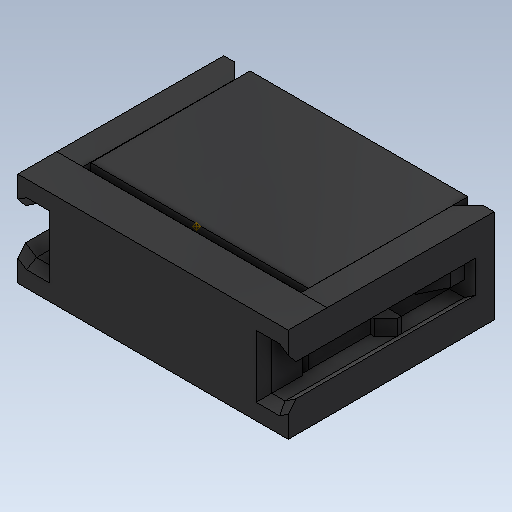
# Autodesk Inventor part: ribbon cable connector
Saved by Autodesk Inventor 2020.1 (Build 241239000, 239)
## iProperties
Created: 2007-05-08
Part Number: ribbon cable connector
Document SubType Name: Modeling
Designer: floress
Density: 1 g/cm^3
Categories: <MemberInstance><Categories><Category DisplayName="" Mnemonic="CABLEANDHARNESS" InternalName="e4a7e005-5e42-4d16-b293-125e7f0d0512"><Category DisplayName="" Mnemonic="CONNECTORS" InternalName="6f634eba-a678-4820-a31d-2c2d5ee6728e"><CategoryParameter DisplayName="" Mnemonic="REFDES" InternalName="c3740e8c-60ab-4d5d-8584-52b73222f2f0"/><Category DisplayName="" Mnemonic="RIBBONCABLE" InternalName="27621a3d-53ec-49ed-8225-e2ac65e8eb52"/></Category></Category></Categories><FamilyTemplate><FamilyTemplateParameters></FamilyTemplateParameters></FamilyTemplate><CategoryParameterMap><ParamToTemplateMap><ParamToTemplate CategoryParameter="//CategoryParameter[@InternalName='c3740e8c-60ab-4d5d-8584-52b73222f2f0']" ConstantValue=""/></ParamToTemplateMap></CategoryParameterMap></MemberInstance>
Material: Generic
Appearance: Dark Gray
Author: floress
Autodesk Inventor part; units mm, degrees
ref_plane "YZ Plane" through (0, 0, 0) normal (1, 0, 0) x (0, 1, 0)
ref_plane "XZ Plane" through (0, 0, 0) normal (0, 1, 0) x (-1, 0, 0)
sketch "Sketch1" plane through (0, 0, 0) normal (0, 0, 1) x (1, 0, 0)
  line L0 (6.98, -3) -> (-6.98, -3)
  line L1 (-6.23, -1.5) -> (-6.23, -2.1)
  line L2 (-6.98, -3) -> (-6.98, -2.1)
  line L3 (-6.23, -2.1) -> (-6.98, -2.1)
  line L4 (-6.98, -1.5) -> (-6.23, -1.5)
  line L5 (-6.98, -1.5) -> (-6.98, 3)
  line L6 (6.23, 1.5) -> (6.23, 2.1)
  line L7 (6.98, 1.5) -> (6.98, -3)
  line L8 (6.98, 1.5) -> (6.23, 1.5)
  line L9 (6.23, 2.1) -> (6.98, 2.1)
  line L10 (6.98, 3) -> (6.98, 2.1)
  line L11 (0, 3) -> (0, -3) construction
  line L12 (-6.98, 3) -> (6.98, 3)
  point P0 (0, 0)
  point P1 (0, 0)
  constraints: 26 end point, 8 parallel, 3 midpoint, 3 perpendicular, 2 horizontal, 1 coincident
extrude "Extrusion1" add sketch "Sketch1" along normal blind 10.2
sketch "Sketch2" plane through (-6.98, -3, 0) normal (0, -1, 0) x (1, 0, 0)
  line L0 (5.18, 3.6) -> (8.78, 3.6)
  line L1 (8.78, 3.6) -> (8.78, 0.5)
  line L2 (8.28, 0) -> (5.68, 0)
  line L3 (5.18, 0.5) -> (5.18, 3.6)
  line L4 (5.18, 0.5) -> (5.68, 0)
  line L5 (8.78, 0.5) -> (8.28, 0)
  point P0 (6.98, 0)
  constraints: 12 end point, 2 parallel, 1 horizontal, 1 midpoint, 1 perpendicular
extrude "Extrusion2" add sketch "Sketch2" along normal blind 1
sketch "Sketch3" plane through (0, 0, 0) normal (0, 1, 0) x (-1, 0, 0)
  line L0 (-6.98, 3.6) -> (-7.23, 3.6)
  line L1 (-7.98, 2.1) -> (-7.98, 1.22)
  line L2 (-7.98, 1.22) -> (-6.98, 1.22)
  line L3 (-6.98, 1.22) -> (-6.98, 3.6)
  line L4 (6.98, 10.2) -> (-6.98, 10.2)
  line L5 (0, 10.2) -> (0, 0)
  line L6 (-6.98, 0) -> (6.98, 0)
  line L7 (-7.23, 3.6) -> (-7.98, 2.1)
  line L8 (6.98, 3.6) -> (7.23, 3.6)
  line L9 (7.98, 2.1) -> (7.98, 1.22)
  line L10 (7.98, 1.22) -> (6.98, 1.22)
  line L11 (6.98, 1.22) -> (6.98, 3.6)
  line L12 (7.23, 3.6) -> (7.98, 2.1)
  constraints: 26 end point, 5 symmetric about line, 2 midpoint, 2 parallel, 2 perpendicular, 1 horizontal
extrude "Extrusion3" add sketch "Sketch3" along normal mid plane 1
sketch "Sketch4" plane through (0, -0.5, 0) normal (0, -1, 0) x (1, 0, 0)
  line L0 (6.98, 3.6) -> (7.23, 3.6)
  line L1 (6.98, 6.263) -> (7.23, 6.263)
  line L2 (7.98, 5.513) -> (7.98, 5.263)
  line L3 (7.98, 5.263) -> (6.98, 5.263)
  line L4 (6.98, 5.263) -> (6.98, 6.263)
  line L5 (-6.98, 10.2) -> (6.98, 10.2)
  line L6 (7.23, 6.263) -> (7.98, 5.513)
  line L7 (-6.98, 5.263) -> (-6.98, 6.263)
  line L8 (-6.98, 6.263) -> (-7.23, 6.263)
  line L9 (-7.23, 6.263) -> (-7.98, 5.513)
  line L10 (-7.98, 5.513) -> (-7.98, 5.263)
  line L11 (-7.98, 5.263) -> (-6.98, 5.263)
  point P0 (0, 10.2)
  constraints: 24 end point, 2 parallel, 1 horizontal, 1 midpoint, 1 perpendicular
extrude "Extrusion4" add sketch "Sketch4" along normal blind 1
sketch "Sketch5" plane through (0, 0.5, 0) normal (0, 1, 0) x (1, 0, 0)
  line L0 (7.23, -3.6) -> (6.98, -3.6)
  line L1 (7.23, -6.263) -> (6.98, -6.263)
  line L2 (6.98, -6.263) -> (6.98, -5.263)
  line L3 (6.98, -5.263) -> (7.98, -5.263)
  line L4 (7.98, -5.263) -> (7.98, -5.513)
  line L5 (6.98, -10.2) -> (-6.98, -10.2)
  line L6 (1.3, 0) -> (-1.3, 0)
  line L7 (0, 0) -> (0, -10.2)
  line L8 (7.23, -6.263) -> (7.98, -5.513)
  line L9 (-6.98, -6.263) -> (-6.98, -5.263)
  line L10 (-7.23, -6.263) -> (-6.98, -6.263)
  line L11 (-7.23, -6.263) -> (-7.98, -5.513)
  line L12 (-7.98, -5.263) -> (-7.98, -5.513)
  line L13 (-6.98, -5.263) -> (-7.98, -5.263)
  line L14 (6.98, -3.6) -> (6.98, -1.22)
  line L15 (7.98, -2.1) -> (7.23, -3.6)
  line L16 (7.98, -1.22) -> (7.98, -2.1)
  line L17 (6.98, -1.22) -> (7.98, -1.22)
  dimension "d35" = 1.663
  dimension "d36" = 13.96
  dimension "d37" = 1
  dimension "d38" = 1
  dimension "d39" = 0.25
  dimension "d40" = 0.25
  constraints: 36 end point, 5 symmetric about line, 2 midpoint, 2 parallel, 1 horizontal, 1 perpendicular
  measures "d35" distance between parallel lines of L0 L3
  measures "d36" diameter of L2 L7
  measures "d37" distance of L2.start L2.end
  measures "d38" distance of L2.end L4.start
  measures "d39" distance of L1.start L2.start
  measures "d40" distance of L4.start L8.end
extrude "Extrusion5" add sketch "Sketch5" along normal blind 1 contours L1 L2 L3 L4 L8 | L10 L11 L12 L13 L9
sketch "Sketch6" plane through (-6.98, -3, 10.2) normal (0, -1, 0) x (1, 0, 0)
  line L0 (0.5, -10.2) -> (2.5, -6.7359)
  line L1 (2.5, -6.7359) -> (4.5, -10.2)
  line L2 (0.5, -10.2) -> (4.5, -10.2)
  line L3 (5.68, -10.2) -> (5.18, -9.7)
  line L4 (5.18, -9.7) -> (5.18, -6.6)
  constraints: 10 end point, 2 equal length
extrude "Extrusion6" cut sketch "Sketch6" against normal blind 0.1
sketch "Sketch7" plane through (0, 0, 0) normal (0, 0, -1) x (-1, 0, 0)
  line L0 (6.98, 3) -> (6.98, -1.5)
  line L1 (4.705, 1.645) -> (5.455, 1.645)
  line L2 (5.455, 1.645) -> (5.455, 0.895)
  line L3 (5.455, 0.895) -> (4.705, 0.895)
  line L4 (4.705, 0.895) -> (4.705, 1.645)
  line L5 (4.705, -0.895) -> (5.455, -0.895)
  line L6 (5.455, -0.895) -> (5.455, -1.645)
  line L7 (5.455, -1.645) -> (4.705, -1.645)
  line L8 (4.705, -1.645) -> (4.705, -0.895)
  line L9 (5.08, 0.895) -> (5.08, -0.895) construction
  line L10 (6.48, -2.9) -> (6.48, -3)
  line L11 (6.98, -3) -> (6.48, -3)
  line L12 (6.98, -2.1) -> (6.98, -3)
  line L13 (6.23, -2.1) -> (6.98, -2.1)
  line L14 (6.23, -1.5) -> (6.23, -2.1)
  point P0 (5.08, 0)
  constraints: 30 end point, 7 equal length, 4 parallel, 3 midpoint, 3 perpendicular, 2 horizontal
extrude "Extrusion7" cut sketch "Sketch7" against normal blind 3
chamfer "Chamfer1" distance 0.5 angle 45 8 edges at (-4.705, 1.27, 0) (-5.08, 0.895, 0) (-5.455, 1.27, 0) (-5.08, 1.645, 0) (-4.705, -1.27, 0) (-5.08, -1.645, 0) (-5.455, -1.27, 0) (-5.08, -0.895, 0)
pattern_linear "Rectangular Pattern1" count 5 spacing 2.54 along (1, 0, 0) of "Extrusion7", "Chamfer1"
ref_plane "Work Plane1" through (0, 0, 10.7) normal (0, 0, 1) x (1, 0, 0)
sketch "Sketch8" plane through (0, 0, 10.7) normal (0, 0, 1) x (1, 0, 0)
  line L0 (-7.9608, -1.4995) -> (-7.11, -1.4995)
  line L1 (-8.665, -1.03) -> (-7.9608, -1.4995)
  line L2 (-8.665, -3.03) -> (-8.665, -1.03)
  line L3 (8.665, -3.03) -> (-8.665, -3.03)
  line L4 (-8.665, 3.03) -> (8.665, 3.03)
  line L5 (-7.11, -1.4995) -> (-7.11, 1.4995)
  line L6 (-6.98, 3) -> (6.98, 3)
  line L7 (-6.98, -1.5) -> (-6.98, 3)
  line L8 (-6.23, -1.5) -> (-6.98, -1.5)
  line L9 (-6.23, -2.1) -> (-6.23, -1.5)
  line L10 (-6.98, -2.1) -> (-6.23, -2.1)
  line L11 (-6.98, -3) -> (-6.98, -2.1)
  line L12 (6.98, -3) -> (-6.98, -3)
  line L13 (6.98, 1.5) -> (6.98, -3)
  line L14 (6.23, 1.5) -> (6.98, 1.5)
  line L15 (6.23, 2.1) -> (6.23, 1.5)
  line L16 (6.98, 2.1) -> (6.23, 2.1)
  line L17 (6.98, 3) -> (6.98, 2.1)
  line L18 (0, 3) -> (0, -3)
  line L19 (-8.665, 1.03) -> (-7.9608, 1.4995)
  line L20 (-8.665, 3.03) -> (-8.665, 1.03)
  line L21 (-7.9608, 1.4995) -> (-7.11, 1.4995)
  line L22 (8.665, 3.03) -> (8.665, 1.03)
  line L23 (8.665, 1.03) -> (7.9608, 1.4995)
  line L24 (7.9608, 1.4995) -> (7.11, 1.4995)
  line L25 (7.11, -1.4995) -> (7.11, 1.4995)
  line L26 (7.9608, -1.4995) -> (7.11, -1.4995)
  line L27 (8.665, -1.03) -> (7.9608, -1.4995)
  line L28 (8.665, -3.03) -> (8.665, -1.03)
  point P0 (0, 0)
  point P1 (0, 0)
  point P2 (-8.665, -2.03)
  point P3 (-7.11, 0)
  point P4 (0, 0)
  constraints: 58 end point, 6 symmetric about line, 5 midpoint, 3 parallel, 3 perpendicular, 1 coincident, 1 horizontal, 1 horizontal alignment
extrude "Extrusion8" add sketch "Sketch8" along normal blind 2.5 contours L0 L5 L21 L19 L20 L4 L22 L23 L24 L25 L26 L27 L28 L3 L2 L1 | L6 L18 L12 L11 L10 L9 L8 L7 | L6 L17 L16 L15 L14 L13 L12 L18
sketch "Sketch9" plane through (0, 0, 10.7) normal (0, 0, -1) x (-1, 0, 0)
  line L0 (-8.665, 3.03) -> (-8.665, 1.03)
  line L1 (8.665, 1.03) -> (8.665, 3.03)
  line L2 (7.9608, 1.4995) -> (8.665, 1.03)
  line L3 (7.11, 1.4995) -> (7.9608, 1.4995)
  line L4 (7.9608, -1.4995) -> (7.11, -1.4995)
  line L5 (8.665, -1.03) -> (7.9608, -1.4995)
  line L6 (8.665, -3.03) -> (8.665, -1.03)
  line L7 (-8.665, -1.03) -> (-8.665, -3.03)
  line L8 (-7.9608, -1.4995) -> (-8.665, -1.03)
  line L9 (-7.11, -1.4995) -> (-7.9608, -1.4995)
  line L10 (-7.9608, 1.4995) -> (-7.11, 1.4995)
  line L11 (-8.665, 1.03) -> (-7.9608, 1.4995)
  line L12 (-6.99, 1.51) -> (-6.24, 1.51)
  line L13 (-6.24, 1.51) -> (-6.24, 2.09)
  line L14 (-6.24, 2.09) -> (-6.99, 2.09)
  line L15 (-6.99, 2.09) -> (-6.99, 3.03)
  line L16 (6.99, -2.09) -> (6.24, -2.09)
  line L17 (6.24, -2.09) -> (6.24, -1.51)
  line L18 (6.24, -1.51) -> (6.99, -1.51)
  line L19 (6.99, -3.03) -> (6.99, -2.09)
  line L20 (-7.11, -1.4995) -> (-6.99, -1.4995)
  line L21 (-7.11, 1.4995) -> (-6.99, 1.4995)
  line L22 (-6.99, -3.03) -> (-6.99, -1.4995)
  line L23 (-6.99, 1.4995) -> (-6.99, 1.51)
  line L24 (7.11, 1.4995) -> (6.99, 1.4995)
  line L25 (7.11, -1.4995) -> (6.99, -1.4995)
  line L26 (6.99, -1.51) -> (6.99, -1.4995)
  line L27 (6.99, 1.4995) -> (6.99, 3.03)
  line L28 (-8.665, 3.03) -> (-8.665, 1.03)
  line L29 (-8.665, 1.03) -> (-7.9608, 1.4995)
  line L30 (-7.9608, 1.4995) -> (-7.11, 1.4995)
  line L31 (-7.11, -1.4995) -> (-7.9608, -1.4995)
  line L32 (-7.9608, -1.4995) -> (-8.665, -1.03)
  line L33 (-8.665, -1.03) -> (-8.665, -3.03)
  line L34 (8.665, -3.03) -> (8.665, -1.03)
  line L35 (8.665, -1.03) -> (7.9608, -1.4995)
  line L36 (7.9608, -1.4995) -> (7.11, -1.4995)
  line L37 (7.11, 1.4995) -> (7.9608, 1.4995)
  line L38 (7.9608, 1.4995) -> (8.665, 1.03)
  line L39 (8.665, 1.03) -> (8.665, 3.03)
  line L40 (8.665, -3.03) -> (6.99, -3.03)
  line L41 (-8.665, -3.03) -> (-6.99, -3.03)
  line L42 (-8.665, 3.03) -> (-6.99, 3.03)
  line L43 (6.99, 3.03) -> (8.665, 3.03)
  constraints: 88 end point, 8 parallel, 6 perpendicular, 2 collinear, 2 horizontal
extrude "Extrusion9" add sketch "Sketch9" along normal blind 10.7
sketch "Sketch10" plane through (0, 0, 0) normal (0, 1, 0) x (-1, 0, 0)
  line L0 (-8.665, 0) -> (-6.99, 0)
  line L1 (-6.99, 0) -> (-6.99, 1.21)
  line L2 (-6.99, 1.21) -> (-8.665, 1.21)
  line L3 (-8.665, 1.21) -> (-8.665, 0)
  line L4 (6.99, 0) -> (6.99, 1.21)
  line L5 (6.99, 1.21) -> (8.665, 1.21)
  line L6 (8.665, 1.21) -> (8.665, 0)
  line L7 (8.665, 0) -> (6.99, 0)
  constraints: 16 end point, 2 parallel, 1 horizontal, 1 perpendicular
extrude "Extrusion10" add sketch "Sketch10" along normal mid plane 6.06
chamfer "Chamfer2" distance 1 angle 45 4 edges at (6.99, 2.56, 0) (6.99, -0.76, 0) (-6.99, 0.76, 0) (-6.99, -2.56, 0)
chamfer "Chamfer3" distance 1.749 angle 45 2 edges at (-6.24, -1.8, 0) (6.24, 1.8, 0)
chamfer "Chamfer4" distance 10.71 distance2 0.03 1 edges at (8.3275, -3.03, 0) measured on face at (2.33, -3.03, 12.3667)
chamfer "Chamfer5" distance 10.71 distance2 0.03 1 edges at (8.3275, 3.03, 0) measured on face at (2.33, 3.03, 12.3667)
chamfer "Chamfer6" distance 0.5 angle 45 10 edges at (-8.3129, 1.2647, 13.2) (-7.5354, 1.4995, 13.2) (-7.11, 0, 13.2) (-7.5354, -1.4995, 13.2) (-8.3129, -1.2647, 13.2) (7.5354, 1.4995, 13.2) (7.11, 0, 13.2) (7.5354, -1.4995, 13.2) (8.3129, -1.2647, 13.2) (8.3129, 1.2647, 13.2)
sketch "Sketch11" plane through (-8.665, -3.03, 13.2) normal (0, -1, 0) x (1, 0, 0)
  point P0 (2.95, -2.75)
sketch "Sketch12" plane through (-8.665, -3.03, 13.2) normal (0, -1, 0) x (1, 0, 0)
  point P0 (8.665, -2.75)
sketch "Sketch13" plane through (-8.665, 3.03, 13.2) normal (0, 1, 0) x (1, 0, 0)
  point P0 (8.665, 2.75)
equation "\"d36\" = d41"
equation "\"d9\" = 13.96"
equation "\"d25\" = 13.96"
equation "\"d41\" = 13.96"
equation "\"d66\" = 17.33"
equation "\"d111\" = 17.33"
body "Solid1"
